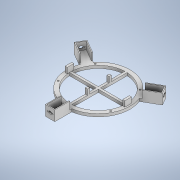
# Autodesk Inventor part: bottom2
Saved by Autodesk Inventor 2020 (Build 240168000, 168)
## iProperties
Created: 2020-03-22
Part Number: bottom2
Material: Generic
Document SubType Name: Modeling
Designer: Tarsoly
Density: 1 g/cm^3
Appearance: Default
Author: Tarsoly
Autodesk Inventor part; units mm, degrees
ref_plane "YZ Plane" through (0, 0, 0) normal (1, 0, 0) x (0, 1, 0)
ref_plane "XZ Plane" through (0, 0, 0) normal (0, 1, 0) x (-1, 0, 0)
ref_plane "XY Plane" through (0, 0, 0) normal (0, 0, 1) x (1, 0, 0)
sketch "Sketch1" plane through (0, 0, 0) normal (0, 1, 0) x (-1, 0, 0)
  circle A0 centre (0, 0) radius 57
  circle A1 centre (0, 0) radius 50
  line L0 (0, -85.8) -> (0, 115.8) projected
  line L1 (111.4319, 0) -> (-111.4319, 0) projected
  line L2 (-50, 2) -> (50, 2)
  line L3 (50, 2) -> (50, -2)
  line L4 (50, -2) -> (-50, -2)
  line L5 (-50, -2) -> (-50, 2)
  line L6 (-50, 2) -> (50, -2) construction
  line L7 (50, 2) -> (-50, -2) construction
  line L8 (2, 50) -> (-2, 50)
  line L9 (-2, 50) -> (-2, -50)
  line L10 (-2, -50) -> (2, -50)
  line L11 (2, -50) -> (2, 50)
  line L12 (2, 50) -> (-2, -50) construction
  line L13 (-2, 50) -> (2, -50) construction
  line L14 (8.5, 87) -> (-8.5, 87)
  line L15 (-8.5, 87) -> (-8.5, 50)
  line L16 (-8.5, 50) -> (8.5, 50)
  line L17 (8.5, 50) -> (8.5, 87)
  line L18 (0, 87) -> (0, 50) construction
  line L19 (8.5, 60) -> (-8.5, 60)
  line L20 (-44.3013, -23.2679) -> (-42.3013, -26.7321)
  line L21 (-39.0513, -32.3612) -> (-47.5513, -17.6388)
  line L22 (-56.2115, -22.6388) -> (-47.7115, -37.3612)
  line L23 (-71.0942, -50.8612) -> (-39.0513, -32.3612)
  line L24 (-47.5513, -17.6388) -> (-79.5942, -36.1388)
  line L25 (-75.3442, -43.5) -> (-43.3013, -25) construction
  line L26 (-79.5942, -36.1388) -> (-71.0942, -50.8612)
  line L27 (42.3013, -26.7321) -> (44.3013, -23.2679)
  line L28 (47.5513, -17.6388) -> (39.0513, -32.3612)
  line L29 (47.7115, -37.3612) -> (56.2115, -22.6388)
  line L30 (79.5942, -36.1388) -> (47.5513, -17.6388)
  line L31 (39.0513, -32.3612) -> (71.0942, -50.8612)
  line L32 (75.3442, -43.5) -> (43.3013, -25) construction
  line L33 (71.0942, -50.8612) -> (79.5942, -36.1388)
  circle A2 centre (0, 0) radius 53.5 construction
  circle A3 centre (40.4629, -35) radius 1.5
  circle A4 centre (-40.4629, -35) radius 1.5
  circle A5 centre (-47.2996, 25) radius 1.5
  circle A6 centre (47.2996, 25) radius 1.5
  point P0 (2, -49.96)
  point P1 (2, -2)
  point P2 (49.96, -2)
  point P3 (-2, 49.96)
  point P4 (-2, 2)
  point P5 (-49.96, 2)
  point P6 (-2, -49.96)
  point P7 (-49.96, -2)
  point P8 (-2, -2)
  point P9 (-8.5, 56.3627)
  point P10 (-53.0615, -20.8201)
  point P11 (-44.5615, -35.5425)
  point P12 (44.5615, -35.5425)
  point P13 (53.0615, -20.8201)
  point P14 (8.5, 56.3627)
  point P15 (2, 49.96)
  point P16 (49.96, 2)
  point P17 (2, 2)
  dimension "d0" = 114
  dimension "d1" = 100
  dimension "d6" = 100
  dimension "d7" = 4
  dimension "d8" = 4
  dimension "d9" = 100
  dimension "d10" = 17
  dimension "d14" = 60
  dimension "d15" = 27
  dimension "d18" = 360
  dimension "d61" = 107
  dimension "d62" = 3
  dimension "d63" = 3
  dimension "d64" = 3
  dimension "d65" = 3
  dimension "d66" = 35
  dimension "d67" = 35
  dimension "d68" = 25
  dimension "d69" = 25
  constraints: 64 end point, 7 centre point, 6 midpoint, 6 parallel, 6 point on line, 4 perpendicular, 4 point on circle, 3 coincident, 3 horizontal, 1 collinear, 1 tangent, 52 other
  measures "d0" diameter of A0
  measures "d1" diameter of A1
  measures "d6" distance of L3.end L4.end
  measures "d7" distance of L2.end L3.end
  measures "d8" distance of L10.end L9.end
  measures "d9" distance of L9.end L8.end
  measures "d10" distance of L16.end L15.end
  measures "d14" distance between parallel lines of L1 L19
  measures "d15" distance between parallel lines of L19 L14
  measures "d61" diameter of A2
  measures "d62" diameter of A3
  measures "d63" diameter of A4
  measures "d64" diameter of A5
  measures "d65" diameter of A6
  measures "d66" distance from line of L1 A3.centre
  measures "d67" distance from line of L1 A4.centre
  measures "d68" distance from line of L1 A5.centre
  measures "d69" distance from line of L1 A6.centre
extrude "Extrusion1" add sketch "Sketch1" along normal blind 5 contours L1 L3 L2 A1 L11 L16 L17 A0 | A0 L30 L28 L27 A1 L4 L3 L1 | L17 L16 L8 L0 A0 | A0 L0 L19 L17 | L30 L29 L31 A0 | A0 L31 L28 L27 L30 | L1 L11 L2 A1 | L3 L4 A1 | A1 L4 L11 L1 | A1 L2 L3 | L0 L8 L16 L15 A0 | A0 L15 L19 L0 | L19 L0 L14 L17 | A0 L0 L10 L11 A1 L27 L28 L31 | L30 L33 L31 L29 | L11 L4 L0 L1 | L1 L0 L2 L11 | L15 L16 L9 A1 L2 L5 L1 A0 | L8 L11 A1 | L0 L2 L9 A1 | A1 L11 L2 L0 | A1 L9 L8 | L19 L15 L14 L0 | A0 L23 L21 L20 A1 L9 L10 L0 | L11 A1 L0 L4 | L1 L9 L2 L0 | L0 L4 L9 L1 | L1 L5 L4 A1 L20 L21 L24 A0 | L23 L22 L24 A0 | A0 L24 L21 L20 L23 | L10 L9 A1 | A1 L9 L4 L0 | A1 L11 L10 | L9 L4 A1 L1 | L1 A1 L2 L9 | L5 L2 A1 | A1 L4 L5 | L23 L26 L24 L22
sketch "Sketch5" plane through (0, 5, 0) normal (0, 1, 0) x (1, 0, 0)
  line L0 (-2, -21.5) -> (2, -21.5)
  line L1 (2, -21.5) -> (2, -17.5)
  line L2 (2, -17.5) -> (-2, -17.5)
  line L3 (-2, -17.5) -> (-2, -21.5)
  line L4 (-2, -2) -> (-2, -49.96) construction
  line L5 (2, -49.96) -> (2, -2) construction
  line L6 (-111.4319, 0) -> (111.4319, 0) construction
  line L7 (-2, 21.5) -> (2, 21.5)
  line L8 (2, 21.5) -> (2, 17.5)
  line L9 (2, 17.5) -> (-2, 17.5)
  line L10 (-2, 17.5) -> (-2, 21.5)
  arc A0 (-49.96, -2) -> (-2, -49.96) centre (0, 0) ccw construction
  arc A1 (-2, 49.96) -> (-49.96, 2) centre (0, 0) ccw construction
  circle A2 centre (0, 0) radius 50 construction
  line L11 (-54, 6) -> (-50, 6)
  line L12 (-50, 6) -> (-50, -6)
  line L13 (-50, -6) -> (-54, -6)
  line L14 (-54, -6) -> (-54, 6)
  line L15 (-54, 0) -> (-50, 0) construction
  line L16 (0, 88.6024) -> (0, -116.2671) construction
  line L17 (54, 6) -> (50, 6)
  line L18 (50, 6) -> (50, -6)
  line L19 (50, -6) -> (54, -6)
  line L20 (54, -6) -> (54, 6)
  line L21 (54, 0) -> (50, 0) construction
  point P0 (49.96, -2)
  point P1 (49.96, 2)
  dimension "d41" = 17.5
  dimension "d42" = 4
  dimension "d43" = 12
  constraints: 36 end point, 12 symmetric about line, 4 parallel, 3 collinear, 3 perpendicular, 2 horizontal, 2 midpoint, 1 centre point, 1 coincident, 1 concentric, 1 tangent
  measures "d41" distance from line of point (0, 0) L2
  measures "d42" distance of L12.end L13.end
  measures "d43" distance of L11.end L12.end
extrude "Extrusion4" add sketch "Sketch5" along normal blind 10
sketch "Sketch6" plane through (0, 5, 0) normal (0, 1, 0) x (1, 0, 0)
  line L0 (-8.5, -87) -> (8.5, -87) projected
  line L1 (8.5, -87) -> (8.5, -56.3627) projected
  line L2 (-8.5, -87) -> (8.5, -87)
  line L3 (8.5, -87) -> (8.5, -60)
  line L4 (8.5, -60) -> (-8.5, -60)
  line L5 (-8.5, -60) -> (-8.5, -87)
  line L6 (-7, -85.5) -> (7, -85.5)
  line L7 (7, -85.5) -> (7, -61.5)
  line L8 (7, -61.5) -> (-7, -61.5)
  line L9 (-7, -61.5) -> (-7, -85.5)
  line L10 (-7, -61.5) -> (-7, -60)
  line L11 (7, -61.5) -> (7, -60)
  point P0 (0, 0)
  dimension "d46" = 27
  dimension "d47" = 1.5
  constraints: 20 end point, 4 parallel, 4 point on line, 3 perpendicular, 1 horizontal, 3 other
  measures "d46" distance between parallel lines of L0 L4
  measures "d47" distance between parallel lines of L5 L9
extrude "Extrusion5" add sketch "Sketch6" along normal blind 13.5 contours L5 L4 L10 L9 L6 L7 L11 L1 L0
sketch "Sketch7" plane through (-8.5, 0, 87) normal (0, 0, 1) x (1, 0, 0)
  line L0 (1.5, 5) -> (15.5, 5) projected
  line L1 (6.5, 5) -> (10.5, 5) projected
  line L2 (8.5, 5) -> (8.5, 10) construction
  circle A0 centre (8.5, 10) radius 2.5
  line L3 (4, 10) -> (8.5, 10) construction
  line L4 (8.5, 10) -> (13, 10) construction
  circle A1 centre (4, 10) radius 1
  circle A2 centre (13, 10) radius 1
  line L5 (4, 11) -> (6.2087, 11)
  line L6 (4, 9) -> (6.2087, 9)
  line L7 (10.7913, 11) -> (13, 11)
  line L8 (10.7913, 9) -> (13, 9)
  point P0 (8.5, 0)
  dimension "d50" = 5
  dimension "d51" = 5
  dimension "d53" = 9
  dimension "d54" = 2
  dimension "d55" = 2
  constraints: 14 end point, 8 point on circle, 4 horizontal, 4 tangent, 3 centre point, 3 coincident, 1 collinear, 1 midpoint, 1 parallel, 1 point on line, 1 vertical
  measures "d50" distance of L2.start L2.end
  measures "d51" diameter of A0
  measures "d53" distance of L4.end L3.start
  measures "d54" diameter of A1
  measures "d55" diameter of A2
extrude "Extrusion6" cut sketch "Sketch7" against normal up to next
pattern_circular "Circular Pattern2" count 3 over 360 about axis through (0, -10, 0) along (0, 1, 0) of "Extrusion6", "Extrusion5"
equation "\"d61\" = 0.5 * d1 + 0.5 * d0"
body "Solid1"
